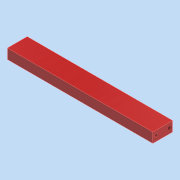
# Autodesk Inventor part: aux_strut
Saved by Autodesk Inventor 2022 (Build 260153000, 153)
## iProperties
Created: 2021-07-29
Part Number: aux_strut
Material: Generic
Document SubType Name: Modeling
Designer: nnico
Density: 1 g/cm^3
Appearance: Red
Author: nnico
Autodesk Inventor part; units mm, degrees
ref_plane "YZ Plane" through (0, 0, 0) normal (1, 0, 0) x (0, 1, 0)
ref_plane "XZ Plane" through (0, 0, 0) normal (0, 1, 0) x (-1, 0, 0)
ref_plane "XY Plane" through (0, 0, 0) normal (0, 0, 1) x (1, 0, 0)
sketch "Sketch1" plane through (0, 0, 0) normal (0, 1, 0) x (-1, 0, 0)
  line L0 (110, -15) -> (-110, -15)
  line L1 (-110, -15) -> (-110, 15)
  line L2 (-110, 15) -> (110, 15)
  line L3 (110, 15) -> (110, -15)
  line L4 (110, 0) -> (-110, 0) construction
  line L5 (0, -15) -> (0, 15) construction
  point P0 (0, 0)
  point P1 (0, 0)
  dimension "d0" = 220
  dimension "d1" = 30
  constraints: 12 end point, 5 midpoint, 2 parallel, 1 coincident, 1 horizontal, 1 perpendicular
  measures "d0" distance of L1.end L2.end
  measures "d1" distance of L2.end L0.start
extrude "Extrusion1" add sketch "Sketch1" along normal blind 15
sketch "Sketch2" plane through (-110, 0, -15) normal (-1, 0, 0) x (0, 0, 1)
  circle A0 centre (5, 7.5) radius 2.5
  line L0 (0, 0) -> (0, 15) construction
  line L1 (0, 7.5) -> (30, 7.5) construction
  line L2 (30, 0) -> (30, 15) construction
  line L3 (15, 0) -> (15, 15) construction
  line L4 (30, 15) -> (0, 15) construction
  circle A1 centre (25, 7.5) radius 2.5
  dimension "d4" = 5
  dimension "d5" = 20
  constraints: 4 end point, 3 midpoint, 2 centre point, 1 point on line, 1 symmetric about line, 1 other
  measures "d4" diameter of A0
  measures "d5" diameter of A0.centre L3
extrude "Extrusion2" cut sketch "Sketch2" against normal blind 8
sketch "Sketch3" plane through (110, 0, 15) normal (1, 0, 0) x (0, 0, -1)
  circle A0 centre (25, 7.5) radius 2.5 projected
  circle A1 centre (5, 7.5) radius 2.5 projected
  point P0 (15, 0)
extrude "Extrusion3" cut sketch "Sketch3" against normal blind 8
body "Solid1"
